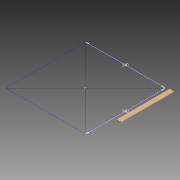
# Autodesk Inventor part: Schalterhalterung
Saved by Autodesk Inventor 2013 SP1 (Build 170176100, 176)
## iProperties
Created: 2012-12-09
Part Number: Schalterhalterung
Material: Platinengrün
Document SubType Name: Modeling
Designer: Sebastian
Density: 1 g/cm^3
Author: Sebastian
Autodesk Inventor part; units mm, degrees
ref_plane "YZ Plane" through (0, 0, 0) normal (1, 0, 0) x (0, 1, 0)
ref_plane "XZ Plane" through (0, 0, 0) normal (0, 1, 0) x (-1, 0, 0)
ref_plane "XY Plane" through (0, 0, 0) normal (0, 0, 1) x (1, 0, 0)
sketch "Skizze Helper" plane through (0, 0, 0) normal (0, 0, 1) x (1, 0, 0)
  line L0 (-170, -170) -> (170, -170) construction
  line L1 (170, -170) -> (170, 170) construction
  line L2 (170, 170) -> (-170, 170) construction
  line L3 (-170, 170) -> (-170, -170) construction
  line L4 (-170, -170) -> (170, 170) construction
  line L5 (170, -170) -> (-170, 170) construction
  point P0 (0, 0)
  dimension "d0" = 340
  dimension "d1" = 340
  constraints: 12 end point, 2 midpoint, 2 parallel, 1 horizontal, 1 perpendicular
  measures "d0" distance of L2.end L1.end
  measures "d1" distance of L1.end L0.end
sketch "Skizze2" plane through (0, 0, 0) normal (0, 0, 1) x (1, 0, 0)
  line L0 (182, 180) -> (201, 180)
  line L1 (201, 180) -> (201, -47)
  line L2 (201, -47) -> (182, -47)
  line L3 (182, -47) -> (182, 180)
  point P0 (0, 0)
  constraints: 8 end point, 2 parallel, 1 horizontal, 1 perpendicular
extrude "Extrusion1" add sketch "Skizze2" against normal blind 2
move or copy body "Körper verschieben1" bodies to move or copy 1 copy no translate (0, 0, -2)
